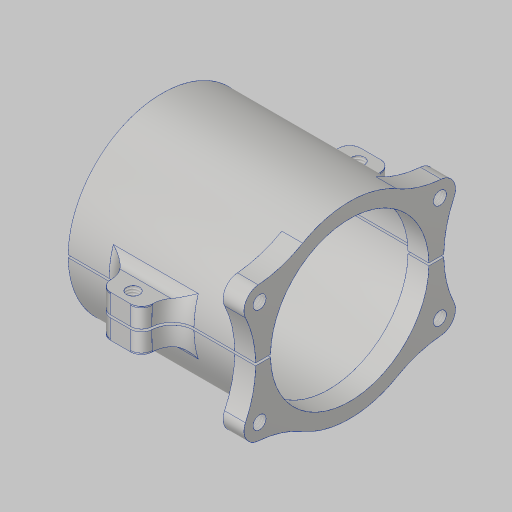
# Autodesk Inventor part: AR-010
Saved by Autodesk Inventor 2023.5 (Build 275446000, 446)
## iProperties
Created: 2025-01-24
Part Number: AR-010
Material: Aluminum 6061
Document SubType Name: Modeling
Designer: slick
Density: 2.7 g/cm^3
Appearance: Aluminum - Flat
Mass: 88.0968 g
Surface Area: 234.144 cm^2
Volume: 32.6284 cm^3
Author: slick
Autodesk Inventor part; units mm, degrees
ref_plane "YZ Plane" through (0, 0, 0) normal (1, 0, 0) x (0, 1, 0)
ref_plane "XZ Plane" through (0, 0, 0) normal (0, 1, 0) x (-1, 0, 0)
sketch "Sketch1" plane through (0, 0, 0) normal (1, 0, 0) x (0, 1, 0)
  circle A0 centre (0, 0) radius 26.162
  circle A1 centre (0, 0) radius 28.702
  dimension "d0" = 52.324
  dimension "d1" = 2.54
  constraints: 2 centre point, 1 coincident
  measures "d0" diameter of A0
  measures "d1" radial gap between concentric circles of A0 A1
extrude "Extrusion1" add sketch "Sketch1" along normal mid plane 50.8
sketch "Sketch2" plane through (25.4, 0, 0) normal (1, 0, 0) x (0, 0, -1)
  line L0 (38.1, -38.1) -> (-38.1, -38.1) construction
  line L1 (-38.1, -38.1) -> (-38.1, 38.1) construction
  line L2 (-38.1, 38.1) -> (38.1, 38.1) construction
  line L3 (38.1, 38.1) -> (38.1, -38.1) construction
  line L4 (38.1, -38.1) -> (-38.1, 38.1) construction
  line L5 (-38.1, -38.1) -> (38.1, 38.1) construction
  circle A0 centre (0, 0) radius 38.1
  circle A1 centre (0, 0) radius 24.13
  dimension "d4" = 76.2
  dimension "d5" = 76.2
  dimension "d20" = 76.2
  dimension "d42" = 48.26
  constraints: 12 end point, 2 centre point, 2 coincident, 2 midpoint, 2 parallel, 1 horizontal, 1 perpendicular
  measures "d4" distance of L1.end L2.end
  measures "d5" distance of L0.end L1.end
  measures "d20" diameter of A0
  measures "d42" diameter of A1
extrude "Extrusion2" add sketch "Sketch2" along normal blind 6.35
sketch "Sketch3" plane through (31.75, 0, 0) normal (1, 0, 0) x (0, 0, -1)
  circle A0 centre (0, 0) radius 31.75 construction
  point P0 (0, 31.75)
  point P1 (-27.4963, 15.875)
  point P2 (-27.4963, -15.875)
  point P3 (0, -31.75)
  point P4 (27.4963, -15.875)
  point P5 (27.4963, 15.875)
  dimension "d46" = 63.5
  dimension "d11" = 360
  constraints: 2 vertical alignment, 1 coincident, 9 other
hole "Hole1" at (31.75, 31.75, 0) at (31.75, 15.875, 27.4963) at (31.75, -15.875, 27.4963) at (31.75, -31.75, 0) at (31.75, -15.875, -27.4963) at (31.75, 15.875, -27.4963) direction (-1, 0, 0) diameter 3.9624 end through all thread size "10-32 UNF" class "2B" standard "ANSI Unified Screw Threads"
ref_plane "Work Plane2" through (0, 0, 38.1) normal (0, 0, 1) x (1, 0, 0)
sketch "Sketch6" plane through (0, 0, 38.1) normal (0, 0, 1) x (1, 0, 0)
  line L0 (6.35, -6.35) -> (-6.35, -6.35)
  line L1 (-6.35, -6.35) -> (-6.35, 6.35)
  line L2 (-6.35, 6.35) -> (6.35, 6.35)
  line L3 (6.35, 6.35) -> (6.35, -6.35)
  line L4 (6.35, -6.35) -> (-6.35, 6.35) construction
  line L5 (-6.35, -6.35) -> (6.35, 6.35) construction
  point P0 (0, 0)
  dimension "d27" = 12.7
  dimension "d28" = 12.7
  constraints: 12 end point, 2 midpoint, 2 parallel, 1 horizontal, 1 perpendicular
  measures "d27" distance of L1.end L2.end
  measures "d28" distance of L0.end L1.end
extrude "Extrusion4" add sketch "Sketch6" against normal blind 11.43
mirror "Mirror1" about plane through (0, 0, 0) normal (0, 0, 1) of "Extrusion4"
fillet "Fillet1" radius 6.604 4 edges at (-6.35, 0, -28.702) (6.35, 0, -28.702) (-6.35, 0, 28.702) (6.35, 0, 28.702)
fillet "Fillet2" radius 3.302 16 edges at (-9.652, 6.35, 27.9908) (0, 6.35, 27.9908) (9.652, 6.35, 27.9908) (-9.652, 6.35, -27.9908) (0, 6.35, -27.9908) (9.652, 6.35, -27.9908) (9.652, -6.35, -27.9908) (0, -6.35, -27.9908) (-9.652, -6.35, -27.9908) (-9.652, -6.35, 27.9908) (0, -6.35, 27.9908) (9.652, -6.35, 27.9908) (-6.35, 0, -38.1) (6.35, 0, -38.1) (-6.35, 0, 38.1) (6.35, 0, 38.1)
sketch "Sketch7" plane through (-3.048, 6.35, -38.1) normal (0, 1, 0) x (1, 0, 0)
  line L0 (-22.352, -66.0908) -> (-22.352, -63.4797) projected
  line L1 (-22.352, -10.1092) -> (-9.906, -10.1092) projected
  line L2 (-4.7595, -7.5862) -> (10.8555, -7.5862) projected
  line L3 (9.398, -3.302) -> (9.398, -3.3697) projected
  line L4 (0, 0) -> (6.096, 0) projected
  line L5 (-3.302, -3.3697) -> (-3.302, -3.302) projected
  line L6 (-22.352, -63.4797) -> (28.448, -63.4797) projected
  line L7 (28.448, -12.7203) -> (-22.352, -12.7203) projected
  line L8 (-22.352, -12.7203) -> (-22.352, -10.1092) projected
  line L9 (-9.906, -66.0908) -> (-22.352, -66.0908) projected
  line L10 (10.8555, -68.6138) -> (-4.7595, -68.6138) projected
  line L11 (9.398, -72.8303) -> (9.398, -72.898) projected
  line L12 (6.096, -76.2) -> (0, -76.2) projected
  line L13 (-3.302, -72.898) -> (-3.302, -72.8303) projected
  line L14 (16.002, -10.1092) -> (28.448, -10.1092) projected
  line L15 (28.448, -75.6671) -> (28.448, -66.0908) projected
  line L16 (34.798, -75.6671) -> (28.448, -75.6671) projected
  line L17 (28.448, -0.5329) -> (34.798, -0.5329) projected
  line L18 (28.448, -10.1092) -> (28.448, -0.5329) projected
  line L19 (28.448, -66.0908) -> (16.002, -66.0908) projected
  line L20 (6.096, -3.302) -> (0, -3.302) construction
  line L21 (6.096, -72.898) -> (0, -72.898) construction
  line L22 (28.448, -63.4797) -> (28.448, -61.3795) projected
  line L23 (28.448, -61.3795) -> (34.798, -61.3795) projected
  line L24 (34.798, -61.3795) -> (34.798, -75.6671) projected
  line L25 (28.448, -14.8205) -> (28.448, -12.7203) projected
  line L26 (34.798, -14.8205) -> (28.448, -14.8205) projected
  line L27 (34.798, -0.5329) -> (34.798, -14.8205) projected
  line L28 (3.048, -76.2) -> (3.048, -68.6138) construction
  line L29 (10.8555, -68.6138) -> (-4.7595, -68.6138) projected
  line L30 (3.048, 0) -> (3.048, -7.5862) construction
  arc A0 (6.096, -76.2) -> (9.398, -72.898) centre (6.096, -72.898) ccw projected
  arc A1 (-3.302, -72.898) -> (0, -76.2) centre (0, -72.898) ccw projected
  arc A2 (0, 0) -> (-3.302, -3.302) centre (0, -3.302) ccw projected
  arc A3 (9.398, -3.302) -> (6.096, 0) centre (6.096, -3.302) ccw projected
  point P0 (3.048, -38.1)
  point P1 (3.048, -72.4069)
  point P2 (3.048, -3.7931)
  point P3 (3.048, -3.302)
  point P4 (3.048, -72.4069)
  point P5 (3.048, -3.7931)
  constraints: 8 end point, 7 midpoint, 2 coincident, 2 horizontal, 2 vertical alignment, 8 other
hole "Hole2" at (0, 6.35, 34.3069) at (0, 6.35, -34.3069) direction (0, -1, 0) diameter 3.9624 end through all thread size "10-32 UNF" class "2B" standard "ANSI Unified Screw Threads"
sketch "Sketch8" plane through (31.75, 0, 0) normal (1, 0, 0) x (0, 0, -1)
  circle A0 centre (27.4963, -15.875) radius 1.9812 projected
  circle A1 centre (-27.4963, -15.875) radius 1.9812 projected
  circle A2 centre (0, 31.75) radius 1.9812 projected
  circle A3 centre (-27.4963, 15.875) radius 1.9812 projected
  circle A4 centre (0, -31.75) radius 1.9812 projected
  circle A5 centre (27.4963, 15.875) radius 1.9812 projected
  circle A6 centre (0, 0) radius 24.13 projected
  circle A7 centre (0, 0) radius 38.1 projected
  circle A8 centre (0, 31.75) radius 1.9812 construction
  circle A9 centre (0, 31.75) radius 4.7625 construction
  circle A10 centre (27.4963, 15.875) radius 4.7625 construction
  circle A11 centre (27.4963, -15.875) radius 4.7625 construction
  circle A12 centre (0, -31.75) radius 4.7625 construction
  circle A13 centre (-27.4963, -15.875) radius 1.9812 construction
  circle A14 centre (-27.4963, -15.875) radius 4.7625 construction
  circle A15 centre (-27.4963, 15.875) radius 1.9812 construction
  circle A16 centre (-27.4963, 15.875) radius 4.7625 construction
  arc A17 (-27.8901, 20.6212) -> (-3.9134, 34.4641) centre (-30.5726, 52.9532) ccw
  arc A18 (3.9134, 34.4641) -> (27.8901, 20.6212) centre (30.5726, 52.9532) ccw
  circle A19 centre (27.4963, -15.875) radius 1.9812 construction
  circle A20 centre (-27.4963, -15.875) radius 1.9812 construction
  circle A21 centre (0, 31.75) radius 1.9812 construction
  circle A22 centre (-27.4963, 15.875) radius 1.9812 construction
  circle A23 centre (0, -31.75) radius 1.9812 construction
  circle A24 centre (27.4963, 15.875) radius 1.9812 construction
  circle A25 centre (0, 0) radius 24.13 construction
  circle A26 centre (0, 0) radius 38.1 construction
  circle A27 centre (0, 0) radius 28.702 construction
  arc A28 (31.8035, 13.8429) -> (31.8035, -13.8429) centre (61.1451, 0) ccw
  arc A29 (27.8901, -20.6212) -> (3.9134, -34.4641) centre (30.5726, -52.9532) ccw
  arc A30 (-3.9134, -34.4641) -> (-27.8901, -20.6212) centre (-30.5726, -52.9532) ccw
  arc A31 (-31.8035, -13.8429) -> (-31.8035, 13.8429) centre (-61.1451, 0) ccw
  arc A32 (3.9134, 34.4641) -> (-3.9134, 34.4641) centre (0, 31.75) ccw
  circle A33 centre (27.4963, 15.875) radius 1.9812 projected
  arc A34 (31.8035, 13.8429) -> (27.8901, 20.6212) centre (27.4963, 15.875) ccw
  arc A35 (27.8901, -20.6212) -> (31.6024, -13.4623) centre (27.4963, -15.875) ccw
  arc A36 (-3.9134, -34.4641) -> (3.9134, -34.4641) centre (0, -31.75) ccw
  arc A37 (-31.8035, -13.8429) -> (-27.8901, -20.6212) centre (-27.4963, -15.875) ccw
  arc A38 (-27.8901, 20.6212) -> (-31.6024, 13.4623) centre (-27.4963, 15.875) ccw
  point P0 (-31.8035, 13.8429)
  point P1 (31.8035, -13.8429)
  dimension "d43" = 9.525
  constraints: 37 point on circle, 18 centre point, 18 tangent, 12 coincident, 6 equal radius
  measures "d43" diameter of A9
extrude "Extrusion5" cut sketch "Sketch8" against normal up to surface (6.35 mm away) contours A7
sketch "Sketch9" plane through (-25.4, 0, 0) normal (-1, 0, 0) x (0, 0, 1)
  circle A0 centre (0, 31.75) radius 1.9812 construction
  arc A1 (3.9134, 34.4641) -> (14.351, 24.8567) centre (30.5726, 52.9532) ccw projected
  arc A2 (3.9134, 34.4641) -> (-3.9134, 34.4641) centre (0, 31.75) ccw projected
  arc A3 (-14.351, 24.8567) -> (-3.9134, 34.4641) centre (-30.5726, 52.9532) ccw projected
  arc A4 (14.351, 24.8567) -> (-14.351, 24.8567) centre (0, 0) ccw projected
  arc A5 (14.351, -24.8567) -> (3.9134, -34.4641) centre (30.5726, -52.9532) ccw projected
  arc A6 (-14.351, -24.8567) -> (14.351, -24.8567) centre (0, 0) ccw projected
  arc A7 (-3.9134, -34.4641) -> (-14.351, -24.8567) centre (-30.5726, -52.9532) ccw projected
  arc A8 (-3.9134, -34.4641) -> (3.9134, -34.4641) centre (0, -31.75) ccw projected
  circle A9 centre (0, -31.75) radius 1.9812 construction
extrude "Extrusion6" cut sketch "Sketch9" against normal through all
split body "Split1" result two bodies by plane through (0, 0, 0) normal (0, 1, 0) first body at (-6.35, 28.0325, 3.0877)
sketch "Sketch10" plane through (-25.4, 0, -26.162) normal (0, 1, 0) x (1, 0, 0)
  line L0 (-9.2697, -68.5744) -> (60.0697, -68.5744)
  line L1 (60.0697, -68.5744) -> (60.0697, 16.2504)
  line L2 (60.0697, 16.2504) -> (-9.2697, 16.2504)
  line L3 (-9.2697, 16.2504) -> (-9.2697, -68.5744)
  line L4 (-9.2697, -68.5744) -> (60.0697, 16.2504) construction
  line L5 (60.0697, -68.5744) -> (-9.2697, 16.2504) construction
  point P0 (25.4, -26.162)
  constraints: 12 end point, 2 midpoint, 2 parallel, 1 horizontal, 1 perpendicular
extrude "Extrusion7" cut sketch "Sketch10" against normal blind 0.381 bodies 3
sketch "Sketch11" plane through (-25.4, 0, -26.162) normal (0, -1, 0) x (1, 0, 0)
  line L0 (-10.3842, -21.0738) -> (61.1842, -21.0738)
  line L1 (61.1842, -21.0738) -> (61.1842, 73.3978)
  line L2 (61.1842, 73.3978) -> (-10.3842, 73.3978)
  line L3 (-10.3842, 73.3978) -> (-10.3842, -21.0738)
  line L4 (-10.3842, -21.0738) -> (61.1842, 73.3978) construction
  line L5 (61.1842, -21.0738) -> (-10.3842, 73.3978) construction
  point P0 (25.4, 26.162)
  constraints: 12 end point, 2 midpoint, 2 parallel, 1 horizontal, 1 perpendicular
extrude "Extrusion8" cut sketch "Sketch11" against normal blind 0.381 bodies 2
body "Solid2"
body "Solid3"
